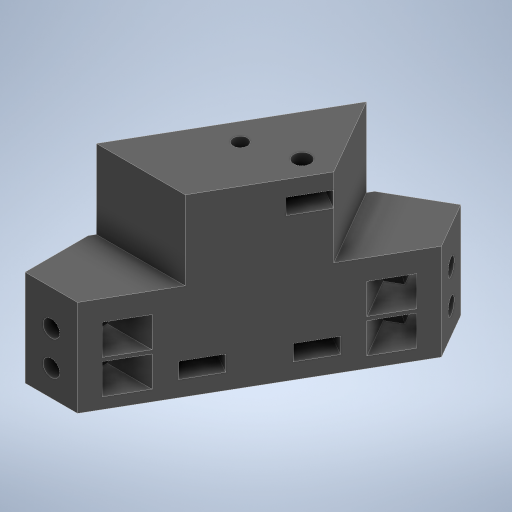
# Autodesk Inventor part: base_plate_towheel
Saved by Autodesk Inventor 2024.1 (Build 281209000, 209)
## iProperties
Created: 2025-02-03
Part Number: base_plate_towheel
Material: 一般
Document SubType Name: モデリング
Designer: hibik
Density: 1 g/cm^3
Appearance: 既定
Sheet Metal Rule: Default_mm
Author: hibik
Autodesk Inventor part; units mm, degrees
ref_plane "YZ Plane" through (0, 0, 0) normal (1, 0, 0) x (0, 1, 0)
ref_plane "XZ Plane" through (0, 0, 0) normal (0, 1, 0) x (-1, 0, 0)
ref_plane "XY Plane" through (0, 0, 0) normal (0, 0, 1) x (1, 0, 0)
sketch "スケッチ1" plane through (0, 0, 0) normal (0, 1, 0) x (-1, 0, 0)
  line L0 (75, 0) -> (105, -51.9615)
  line L1 (-75, 0) -> (-105, -51.9615)
  line L2 (0, -220.136) -> (0, 47.7586) projected
  line L3 (147, 0) -> (-147, 0) projected
  line L4 (37.5, -27) -> (-37.5, -27)
  line L5 (105, -51.9615) -> (30, -181.8653)
  line L6 (30, -181.8653) -> (-30, -181.8653)
  line L7 (-30, -181.8653) -> (-105, -51.9615)
  line L8 (75, 0) -> (-75, 0)
  line L9 (-25.3673, -135.8894) -> (-62.8673, -70.9375)
  line L10 (25.3673, -135.8894) -> (62.8673, -70.9375)
  line L11 (-37.5, -27) -> (-27.5, -27)
  line L12 (-27.5, -27) -> (-27.5, -39)
  line L13 (-27.5, -39) -> (-37.5, -39)
  line L14 (-37.5, -39) -> (-37.5, -27)
  line L15 (37.5, -27) -> (27.5, -27)
  line L16 (27.5, -27) -> (27.5, -39)
  line L17 (27.5, -39) -> (37.5, -39)
  line L18 (37.5, -39) -> (37.5, -27)
  line L19 (0, -77.9423) -> (44.1173, -103.4134) construction
  line L20 (0, -77.9423) -> (-44.1173, -103.4134) construction
  line L21 (-44.1173, -103.4134) -> (-67.5, -116.9134) construction
  line L22 (-57.8673, -79.5977) -> (-47.475, -73.5977)
  line L23 (-52.475, -64.9375) -> (-62.8673, -70.9375)
  line L24 (-62.8673, -70.9375) -> (-57.8673, -79.5977)
  line L25 (-47.475, -73.5977) -> (-52.475, -64.9375)
  line L26 (-25.3673, -135.8894) -> (-30.3673, -127.2291)
  line L27 (-19.975, -121.2291) -> (-14.975, -129.8894)
  line L28 (-14.975, -129.8894) -> (-25.3673, -135.8894)
  line L29 (-30.3673, -127.2291) -> (-19.975, -121.2291)
  line L30 (30.3673, -127.2291) -> (19.975, -121.2291)
  line L31 (14.975, -129.8894) -> (25.3673, -135.8894)
  line L32 (25.3673, -135.8894) -> (30.3673, -127.2291)
  line L33 (19.975, -121.2291) -> (14.975, -129.8894)
  line L34 (62.8673, -70.9375) -> (57.8673, -79.5977)
  line L35 (47.475, -73.5977) -> (52.475, -64.9375)
  line L36 (52.475, -64.9375) -> (62.8673, -70.9375)
  line L37 (57.8673, -79.5977) -> (47.475, -73.5977)
  line L38 (62.8673, -70.9375) -> (37.5, -27)
  line L39 (-37.5, -27) -> (-62.8673, -70.9375)
  line L40 (-25.3673, -135.8894) -> (25.3673, -135.8894)
  line L41 (-27.5, -39) -> (-47.475, -73.5977)
  point P0 (0, 0)
  point P1 (0, 0)
  point P2 (0, -27)
  dimension "d1" = 150
  dimension "d2" = 60
  dimension "d3" = 60
  dimension "d4" = 27
  dimension "d5" = 75
  dimension "d6" = 60
  dimension "d7" = 27
  dimension "d8" = 10
  dimension "d9" = 12
  dimension "d10" = 10
  dimension "d11" = 12
  dimension "d14" = 360
  constraints: 80 end point, 6 equal length, 6 parallel, 4 horizontal, 4 midpoint, 3 coincident, 3 perpendicular, 2 symmetric about line, 1 collinear, 1 horizontal alignment, 1 point on line, 1 vertical alignment, 50 other
  measures "d1" distance of L1.start L0.start
  measures "d2" angle of L3 L0
  measures "d3" angle of L1 L3
  measures "d4" distance between parallel lines of L3 L4
  measures "d5" distance of L4.start L4.end
  measures "d6" distance of L5.end L6.end
  measures "d7" distance between parallel lines of L7 L9
  measures "d8" distance of L12.end L13.end
  measures "d9" distance of L11.end L12.end
  measures "d10" distance of L17.end L16.end
  measures "d11" distance of L16.end L15.end
extrude "押し出し1" add sketch "スケッチ1" along normal blind 18.3 contours L12 L13 L14 L4 | L14 L13 L41 L25 L23 L39 | L23 L25 L22 L9
sketch "スケッチ2" plane through (27.5, 0, -27) normal (0, 0, 1) x (1, 0, 0)
  circle A0 centre (5, 11.5) radius 1.6 projected
  circle A1 centre (5, 5) radius 1.6 projected
  point P0 (-27.5, 0)
sketch "スケッチ3" plane through (27.5, 0, -27) normal (0, 0, 1) x (1, 0, 0)
  circle A0 centre (5, 11.5) radius 1.6 projected
  circle A1 centre (5, 5) radius 1.6 projected
  line L0 (8.3486, 11.5) -> (6.6743, 8.6)
  line L1 (6.6743, 8.6) -> (3.3257, 8.6)
  line L2 (3.3257, 8.6) -> (1.6514, 11.5)
  line L3 (1.6514, 11.5) -> (3.3257, 14.4)
  line L4 (3.3257, 14.4) -> (6.6743, 14.4)
  line L5 (6.6743, 14.4) -> (8.3486, 11.5)
  line L6 (6.6743, 7.9) -> (8.3486, 5)
  line L7 (8.3486, 5) -> (6.6743, 2.1)
  line L8 (6.6743, 2.1) -> (3.3257, 2.1)
  line L9 (3.3257, 2.1) -> (1.6514, 5)
  line L10 (1.6514, 5) -> (3.3257, 7.9)
  line L11 (3.3257, 7.9) -> (6.6743, 7.9)
  point P0 (-27.5, 0)
  dimension "d19" = 5.8
  constraints: 24 end point, 2 coincident, 2 horizontal, 1 parallel, 26 other
  measures "d19" distance from line of L0.end L4
extrude "押し出し2" cut sketch "スケッチ3" against normal blind 6 contours A0 | A1 | L0 L1 L2 L3 L4 L5 | L6 L7 L8 L9 L10 L11
extrude "押し出し3" add sketch "スケッチ3" against normal blind 3
sketch "スケッチ4" plane through (27.5, 0, -33) normal (0, 0, 1) x (1, 0, 0)
  line L0 (3.3257, 14.4) -> (6.6743, 14.4)
  line L1 (1.6514, 11.5) -> (3.3257, 14.4)
  line L2 (3.3257, 8.6) -> (1.6514, 11.5)
  line L3 (6.6743, 8.6) -> (3.3257, 8.6)
  line L4 (1.6514, 5) -> (3.3257, 7.9)
  line L5 (3.3257, 2.1) -> (1.6514, 5)
  line L6 (6.6743, 2.1) -> (3.3257, 2.1)
  line L7 (3.3257, 7.9) -> (6.6743, 7.9)
  line L8 (3.3257, 14.4) -> (6.6743, 14.4) projected
  line L9 (6.6743, 14.4) -> (42.8332, 14.4)
  line L10 (42.8332, 14.4) -> (42.8332, 8.6)
  line L11 (42.8332, 8.6) -> (6.6743, 8.6)
  line L12 (6.6743, 7.9) -> (42.8332, 7.9)
  line L13 (42.8332, 7.9) -> (42.8332, 2.1)
  line L14 (42.8332, 2.1) -> (6.6743, 2.1)
  line L15 (6.6743, 7.9) -> (3.3257, 7.9) projected
  line L16 (3.3257, 2.1) -> (6.6743, 2.1) projected
  line L17 (1.6514, 5) -> (3.3257, 2.1) projected
  line L18 (3.3257, 7.9) -> (1.6514, 5) projected
  line L19 (3.3257, 8.6) -> (6.6743, 8.6) projected
  line L20 (1.6514, 11.5) -> (3.3257, 8.6) projected
  line L21 (3.3257, 14.4) -> (1.6514, 11.5) projected
  point P0 (-27.5, 0)
  constraints: 28 end point, 4 collinear, 2 horizontal, 2 parallel, 2 perpendicular, 2 point on line
extrude "押し出し4" cut sketch "スケッチ4" along normal blind 3
sketch "スケッチ5" plane through (62.8673, 0, -70.9375) normal (0.8660254, 0, 0.5) x (0.5, 0, -0.8660254)
  line L0 (-5.3923, 18.3) -> (-45.3423, 18.3) projected
  line L1 (-25.3673, 18.3) -> (-25.3673, 0)
  line L2 (-5.3923, 0) -> (-45.3423, 0) projected
  point P0 (-92.8673, 0)
  constraints: 2 end point, 2 midpoint
ref_plane "作業平面1" through (50.1837, 18.3, -48.9687) normal (-0.5, 0, 0.8660254) x (0, -1, 0)
mirror "ミラー1" about plane through (50.1837, 18.3, -48.9687) normal (-0.5, 0, 0.8660254) of "押し出し2", "押し出し3", "押し出し4"
sketch "スケッチ6" plane through (0, 0, 0) normal (0, -1, 0) x (1, 0, 0)
  line L0 (37.5, -27) -> (62.8673, -70.9375) projected
  circle A0 centre (40.9875, -45.0405) radius 1.6
  line L1 (42.7196, -48.0405) -> (39.2555, -48.0405)
  line L2 (39.2555, -48.0405) -> (37.5234, -45.0405)
  line L3 (37.5234, -45.0405) -> (39.2555, -42.0405)
  line L4 (39.2555, -42.0405) -> (42.7196, -42.0405)
  line L5 (42.7196, -42.0405) -> (44.4516, -45.0405)
  line L6 (44.4516, -45.0405) -> (42.7196, -48.0405)
  line L7 (50.1837, -48.9687) -> (37.4875, -56.2989)
  line L8 (47.475, -73.5977) -> (27.5, -39) projected
  line L9 (37.6966, -45.0405) -> (39.3421, -42.1905)
  line L10 (39.3421, -42.1905) -> (42.633, -42.1905)
  line L11 (42.633, -42.1905) -> (44.2784, -45.0405)
  line L12 (44.2784, -45.0405) -> (42.633, -47.8905)
  line L13 (42.633, -47.8905) -> (39.3421, -47.8905)
  line L14 (39.3421, -47.8905) -> (37.6966, -45.0405)
  point P0 (0, 0)
  dimension "d27" = 3.2
  dimension "d29" = 6
  dimension "d30" = 6
  dimension "d31" = 8
  dimension "d32" = 5.7
  constraints: 26 end point, 2 coincident, 2 midpoint, 2 parallel, 1 centre point, 26 other
  measures "d27" diameter of A0
  measures "d29" distance between parallel lines of L2 L5
  measures "d30" distance from line of L0 A0.centre
  measures "d31" distance from line of L7 A0.centre
  measures "d32" distance between parallel lines of L14 L11
extrude "押し出し5" cut sketch "スケッチ6" against normal through all contours A0 | L1 L2 L3 L4 L5 L6 | L9 L10 L11 L12 L13 L14
extrude "押し出し6" add sketch "スケッチ6" against normal blind 6 contours L1 L2 L3 L4 L5 L6
extrude "押し出し7" add sketch "スケッチ6" against normal blind 3 contours L9 L10 L11 L12 L13 L14
mirror "ミラー2" about plane through (50.1837, 18.3, -48.9687) normal (-0.5, 0, 0.8660254) of "押し出し5", "押し出し6", "押し出し7"
sketch "スケッチ8" plane through (0, 6, 0) normal (0, 1, 0) x (1, 0, 0)
  line L0 (47.2555, 55.8969) -> (45.5234, 58.8969) projected
  line L1 (45.5234, 58.8969) -> (47.2555, 61.8969) projected
  line L2 (47.2555, 61.8969) -> (50.7196, 61.8969) projected
  line L3 (50.7196, 61.8969) -> (52.4516, 58.8969) projected
  line L4 (52.4516, 58.8969) -> (50.7196, 55.8969) projected
  line L5 (50.7196, 55.8969) -> (47.2555, 55.8969) projected
  line L6 (42.7196, 42.0405) -> (39.2555, 42.0405) projected
  line L7 (39.2555, 42.0405) -> (37.5234, 45.0405) projected
  line L8 (37.5234, 45.0405) -> (39.2555, 48.0405) projected
  line L9 (39.2555, 48.0405) -> (42.7196, 48.0405) projected
  line L10 (42.7196, 48.0405) -> (44.4516, 45.0405) projected
  line L11 (44.4516, 45.0405) -> (42.7196, 42.0405) projected
  line L12 (57.8673, 79.5977) -> (47.475, 73.5977) projected
  line L13 (47.475, 73.5977) -> (27.5, 39) projected
  line L14 (27.5, 39) -> (27.5, 27) projected
  line L15 (27.5, 27) -> (37.5, 27) projected
  line L16 (37.5, 27) -> (62.8673, 70.9375) projected
  line L17 (62.8673, 70.9375) -> (57.8673, 79.5977) projected
  point P0 (0, 0)
extrude "押し出し8" add sketch "スケッチ8" along normal up to surface (12.3 mm away) contours L0 L1 L2 L3 L4 L5 | L6 L7 L8 L9 L10 L11
sketch "スケッチ9" plane through (0, 6, 0) normal (0, -1, 0) x (1, 0, 0)
  line L0 (42.633, -42.1905) -> (39.3421, -42.1905) projected
  line L1 (39.3421, -42.1905) -> (37.6966, -45.0405) projected
  line L2 (37.6966, -45.0405) -> (39.3421, -47.8905) projected
  line L3 (39.3421, -47.8905) -> (42.633, -47.8905) projected
  line L4 (42.633, -47.8905) -> (44.2784, -45.0405) projected
  line L5 (44.2784, -45.0405) -> (42.633, -42.1905) projected
  line L6 (52.2784, -58.8969) -> (50.633, -61.7469) projected
  line L7 (50.633, -56.0469) -> (52.2784, -58.8969) projected
  line L8 (47.3421, -56.0469) -> (50.633, -56.0469) projected
  line L9 (45.6966, -58.8969) -> (47.3421, -56.0469) projected
  line L10 (47.3421, -61.7469) -> (45.6966, -58.8969) projected
  line L11 (50.633, -61.7469) -> (47.3421, -61.7469) projected
  line L12 (42.633, -47.8905) -> (47.8291, -44.8905)
  line L13 (37.5, -27) -> (62.8673, -70.9375) projected
  line L14 (39.3421, -42.1905) -> (44.5382, -39.1905)
  line L15 (47.3421, -56.0469) -> (52.5382, -53.0469)
  line L16 (50.633, -61.7469) -> (55.8291, -58.7469)
  point P0 (0, 0)
  constraints: 8 end point, 4 point on line, 3 perpendicular, 1 parallel
extrude "押し出し9" cut sketch "スケッチ9" along normal blind 3
sketch "スケッチ10" plane through (0, 18.3, 0) normal (0, 1, 0) x (1, 0, 0)
  line L0 (47.475, 73.5977) -> (27.5, 39) projected
  line L1 (28.0774, 40) -> (45.0056, 40)
  line L2 (44.5382, 39.1905) -> (47.8291, 44.8905) projected
  line L3 (46.8977, 72.5977) -> (55.3618, 57.9375)
  line L4 (37.5, 27) -> (62.8673, 70.9375) projected
  line L5 (27.5, 27) -> (37.5, 27) projected
  line L6 (62.8673, 70.9375) -> (57.8673, 79.5977) projected
  point P0 (0, 0)
  dimension "d43" = 1
  dimension "d44" = 1
  constraints: 4 end point, 4 point on line, 2 parallel
  measures "d43" distance from line of L0.end L1
  measures "d44" distance from line of L0.start L3
extrude "押し出し10" add sketch "スケッチ10" along normal blind 15
sketch "スケッチ11" plane through (0, 33.3, 0) normal (0, 1, 0) x (1, 0, 0)
  circle A0 centre (43.2196, 44.9066) radius 1.6 projected
  circle A1 centre (50.2196, 57.0309) radius 1.6 projected
  line L0 (46.5105, 44.9066) -> (44.865, 42.0566)
  line L1 (44.865, 42.0566) -> (41.5741, 42.0566)
  line L2 (41.5741, 42.0566) -> (39.9287, 44.9066)
  line L3 (39.9287, 44.9066) -> (41.5741, 47.7566)
  line L4 (41.5741, 47.7566) -> (44.865, 47.7566)
  line L5 (44.865, 47.7566) -> (46.5105, 44.9066)
  line L6 (53.5105, 57.0309) -> (51.865, 54.1809)
  line L7 (51.865, 54.1809) -> (48.5741, 54.1809)
  line L8 (48.5741, 54.1809) -> (46.9287, 57.0309)
  line L9 (46.9287, 57.0309) -> (48.5741, 59.8809)
  line L10 (48.5741, 59.8809) -> (51.865, 59.8809)
  line L11 (51.865, 59.8809) -> (53.5105, 57.0309)
  line L12 (46.8977, 72.5977) -> (28.0774, 40) projected
  line L13 (41.5741, 42.0566) -> (45.0382, 40.0566)
  line L14 (44.865, 47.7566) -> (48.3291, 45.7566)
  line L15 (45.0056, 40) -> (55.3618, 57.9375) projected
  line L16 (48.5741, 54.1809) -> (52.0382, 52.1809)
  line L17 (51.865, 59.8809) -> (55.3291, 57.8809)
  line L18 (55.8291, 58.7469) -> (52.5382, 53.0469) projected
  point P0 (0, 0)
  dimension "d47" = 5.7
  constraints: 32 end point, 4 perpendicular, 4 point on line, 2 coincident, 2 parallel, 1 collinear, 26 other
  measures "d47" distance between parallel lines of L0 L3
extrude "押し出し11" cut sketch "スケッチ11" against normal blind 6 contours A1 | L11 L17 L15 L16 L7 L6 | L6 L7 L8 L9 L10 L11
sketch "スケッチ13" plane through (0, 33.3, 0) normal (0, 1, 0) x (1, 0, 0)
  circle A0 centre (50.2196, 57.0309) radius 1.6 projected
  circle A1 centre (43.2196, 44.9066) radius 1.6 projected
  line L0 (55.3618, 57.9375) -> (45.0056, 40) projected
  line L1 (55.3618, 57.9375) -> (46.8977, 72.5977) projected
  line L2 (45.0056, 40) -> (28.0774, 40) projected
  line L3 (46.8977, 72.5977) -> (28.0774, 40) projected
  point P0 (0, 0)
extrude "押し出し12" add sketch "スケッチ13" against normal blind 3
sketch "スケッチ15" plane through (0, 0, 0) normal (0, -1, 0) x (1, 0, 0)
  circle A0 centre (40.9875, -45.0405) radius 1.6 projected
  point P0 (0, 0)
extrude "押し出し14" cut sketch "スケッチ15" against normal blind 15
sketch "スケッチ16" plane through (0, 33.3, 0) normal (0, 1, 0) x (1, 0, 0)
  circle A0 centre (41.5234, 53.9687) radius 1.6 projected
  circle A1 centre (41.5234, 53.9687) radius 1.35
  point P0 (0, 0)
  dimension "d56" = 2.7
  constraints: 1 centre point, 1 coincident
  measures "d56" diameter of A1
extrude "押し出し15" cut sketch "スケッチ16" against normal blind 15 contours A1
sketch "スケッチ17" plane through (27.5, 0, -27) normal (0, 0, 1) x (1, 0, 0)
  circle A0 centre (5, 11.5) radius 1.6 projected
  circle A1 centre (5, 5) radius 1.6 projected
  point P0 (-27.5, 0)
extrude "押し出し16" cut sketch "スケッチ17" against normal blind 15
sketch "スケッチ18" plane through (27.5, 0, -33) normal (0, 0, 1) x (1, 0, 0)
  line L0 (11.7321, 14.4) -> (3.3257, 14.4) projected
  line L1 (11.7321, 8.6) -> (11.7321, 14.4) projected
  line L2 (3.3257, 8.6) -> (11.7321, 8.6) projected
  line L3 (1.6514, 11.5) -> (3.3257, 8.6) projected
  line L4 (3.3257, 14.4) -> (1.6514, 11.5) projected
  circle A0 centre (5, 11.5) radius 1.6 projected
  line L5 (3.3257, 7.9) -> (1.6514, 5) projected
  line L6 (11.7321, 7.9) -> (3.3257, 7.9) projected
  line L7 (11.7321, 2.1) -> (11.7321, 7.9) projected
  line L8 (3.3257, 2.1) -> (11.7321, 2.1) projected
  line L9 (1.6514, 5) -> (3.3257, 2.1) projected
  circle A1 centre (5, 5) radius 1.6 projected
  circle A2 centre (5, 11.5) radius 1.6 projected
  line L10 (3.3257, 14.4) -> (1.6514, 11.5) projected
  line L11 (3.3257, 14.4) -> (6.6743, 14.4)
  line L12 (6.6743, 14.4) -> (8.3486, 11.5)
  line L13 (8.3486, 11.5) -> (6.6743, 8.6)
  line L14 (6.6743, 8.6) -> (3.3257, 8.6)
  line L15 (3.3257, 8.6) -> (1.6514, 11.5)
  line L16 (1.6514, 11.5) -> (3.3257, 14.4)
  line L17 (3.3257, 7.9) -> (6.6743, 7.9)
  line L18 (6.6743, 7.9) -> (8.3486, 5)
  line L19 (8.3486, 5) -> (6.6743, 2.1)
  line L20 (6.6743, 2.1) -> (3.3257, 2.1)
  line L21 (3.3257, 2.1) -> (1.6514, 5)
  line L22 (1.6514, 5) -> (3.3257, 7.9)
  circle A3 centre (5, 11.5) radius 1.6 projected
  line L23 (13.4641, 14.4) -> (3.3257, 14.4) projected
  line L24 (1.6514, 11.5) -> (3.3257, 14.4) projected
  line L25 (3.3257, 8.6) -> (1.6514, 11.5) projected
  line L26 (13.4641, 8.6) -> (3.3257, 8.6) projected
  line L27 (13.4641, 14.4) -> (13.4641, 8.6) projected
  circle A4 centre (5, 5) radius 1.6 projected
  line L28 (1.6514, 5) -> (3.3257, 7.9) projected
  line L29 (3.3257, 2.1) -> (1.6514, 5) projected
  line L30 (13.4641, 2.1) -> (3.3257, 2.1) projected
  line L31 (13.4641, 7.9) -> (13.4641, 2.1) projected
  line L32 (13.4641, 7.9) -> (3.3257, 7.9) projected
  line L33 (13.4641, 14.4) -> (3.3257, 14.4) projected
  line L34 (13.4641, 14.4) -> (19.9095, 14.4)
  line L35 (19.9095, 14.4) -> (19.9095, 8.6)
  line L36 (19.9095, 8.6) -> (13.4641, 8.6)
  line L37 (13.4641, 8.6) -> (13.4641, 14.4)
  line L38 (13.4641, 7.9) -> (20.4427, 7.9)
  line L39 (20.4427, 7.9) -> (20.4427, 2.1)
  line L40 (20.4427, 2.1) -> (13.4641, 2.1)
  line L41 (13.4641, 2.1) -> (13.4641, 7.9)
  line L42 (13.4641, 2.1) -> (11.7321, 2.1) projected
  line L43 (13.4641, 8.6) -> (11.7321, 8.6) projected
  point P0 (-27.5, 0)
  point P1 (6.6743, 2.1)
  point P2 (6.6743, 7.9)
  point P3 (6.6743, 8.6)
  point P4 (6.6743, 14.4)
  constraints: 40 end point, 4 parallel, 2 coincident, 2 collinear, 2 horizontal, 2 perpendicular, 26 other
extrude "押し出し17" cut sketch "スケッチ18" against normal blind 3 contours L1 L2 L13 L12 L0 | L23 L27 L26 L1 | L34 L35 L36 L27 | L6 L7 L8 L19 L18 | L32 L31 L30 L7 | L38 L39 L40 L31
mirror "ミラー4" about plane through (50.1837, 18.3, -48.9687) normal (-0.5, 0, 0.8660254) of "押し出し14", "押し出し16", "押し出し17"
equation "\"d3\" = d2"
equation "\"d7\" = d4"
equation "\"BendRadius\" = Thickness"
equation "\"BendReliefWidth\" = Thickness"
equation "\"BendReliefDepth\" = 0.5 * Thickness"
equation "\"CornerReliefSize\" = 4 * Thickness"
equation "\"MinimumRemnant\" = 2 * Thickness"
equation "\"TransitionRadius\" = BendRadius"
equation "\"JacobiRadiusSize\" = BendRadius"
equation "\"GapSize\" = Thickness"
equation "\"Thickness\" = 1.5"
